Autodesk Inventor part; units mm, degrees
(part 2 of 2)
  line L496 (6.7661, -13.5845) -> (6.8293, -13.6645) construction
  line L497 (6.8293, -13.6645) -> (6.8259, -13.7023) construction
  line L498 (6.8259, -13.7023) -> (6.8218, -13.747) construction
  line L499 (6.8218, -13.747) -> (6.7624, -13.8212) construction
  line L500 (6.7624, -13.8212) -> (6.7246, -13.8227) construction
  line L501 (6.7246, -13.8227) -> (6.4551, -13.8332) construction
  line L502 (6.4551, -13.8332) -> (6.185, -13.8306) construction
  line L503 (6.185, -13.8306) -> (5.9152, -13.8264) construction
  line L504 (5.9152, -13.8264) -> (5.8753, -13.8258) construction
  line L505 (5.8753, -13.8258) -> (5.8359, -13.7944) construction
  line L506 (5.8359, -13.7944) -> (5.7963, -13.7773) construction
  line L507 (5.7963, -13.7773) -> (5.7963, -13.7286) construction
  line L508 (5.7963, -13.7286) -> (5.7963, -13.68) construction
  line L509 (5.7963, -13.68) -> (5.7963, -13.6313) construction
  spline S21 degree 3 poles (5.7963, -12.2084) (6.1054, -12.1913) (6.4145, -12.17) (6.7238, -12.163) (6.7594, -12.1622) (6.8243, -12.2405) (6.8254, -12.2834) (6.8264, -12.324) (6.7627, -12.4009) (6.7252, -12.4023) (6.4526, -12.4122) (6.1794, -12.409) (5.9065, -12.4044) (5.8695, -12.4037) (5.833, -12.3718) (5.7963, -12.3543) (5.7963, -12.3057) (5.7963, -12.257) (5.7963, -12.2084) knots 0 0 0 0 1 1 1 2 2 2 3 3 3 4 4 4 5 5 5 6 6 6 6
  line L510 (5.7963, -12.2084) -> (6.1054, -12.1913) construction
  line L511 (6.1054, -12.1913) -> (6.4145, -12.17) construction
  line L512 (6.4145, -12.17) -> (6.7238, -12.163) construction
  line L513 (6.7238, -12.163) -> (6.7594, -12.1622) construction
  line L514 (6.7594, -12.1622) -> (6.8243, -12.2405) construction
  line L515 (6.8243, -12.2405) -> (6.8254, -12.2834) construction
  line L516 (6.8254, -12.2834) -> (6.8264, -12.324) construction
  line L517 (6.8264, -12.324) -> (6.7627, -12.4009) construction
  line L518 (6.7627, -12.4009) -> (6.7252, -12.4023) construction
  line L519 (6.7252, -12.4023) -> (6.4526, -12.4122) construction
  line L520 (6.4526, -12.4122) -> (6.1794, -12.409) construction
  line L521 (6.1794, -12.409) -> (5.9065, -12.4044) construction
  line L522 (5.9065, -12.4044) -> (5.8695, -12.4037) construction
  line L523 (5.8695, -12.4037) -> (5.833, -12.3718) construction
  line L524 (5.833, -12.3718) -> (5.7963, -12.3543) construction
  line L525 (5.7963, -12.3543) -> (5.7963, -12.3057) construction
  line L526 (5.7963, -12.3057) -> (5.7963, -12.257) construction
  line L527 (5.7963, -12.257) -> (5.7963, -12.2084) construction
  spline S22 degree 3 poles (10.3388, -17.736) (10.3217, -17.43) (10.2998, -17.124) (10.2933, -16.8177) (10.2925, -16.7792) (10.369, -16.7138) (10.4159, -16.7076) (10.4519, -16.7028) (10.5321, -16.7702) (10.5336, -16.8078) (10.5438, -17.0774) (10.541, -17.3475) (10.5363, -17.6174) (10.5356, -17.6573) (10.5027, -17.6965) (10.4848, -17.736) (10.4361, -17.736) (10.3875, -17.736) (10.3388, -17.736) knots 0 0 0 0 1 1 1 2 2 2 3 3 3 4 4 4 5 5 5 6 6 6 6
  line L528 (10.3388, -17.736) -> (10.3217, -17.43) construction
  line L529 (10.3217, -17.43) -> (10.2998, -17.124) construction
  line L530 (10.2998, -17.124) -> (10.2933, -16.8177) construction
  line L531 (10.2933, -16.8177) -> (10.2925, -16.7792) construction
  line L532 (10.2925, -16.7792) -> (10.369, -16.7138) construction
  line L533 (10.369, -16.7138) -> (10.4159, -16.7076) construction
  line L534 (10.4159, -16.7076) -> (10.4519, -16.7028) construction
  line L535 (10.4519, -16.7028) -> (10.5321, -16.7702) construction
  line L536 (10.5321, -16.7702) -> (10.5336, -16.8078) construction
  line L537 (10.5336, -16.8078) -> (10.5438, -17.0774) construction
  line L538 (10.5438, -17.0774) -> (10.541, -17.3475) construction
  line L539 (10.541, -17.3475) -> (10.5363, -17.6174) construction
  line L540 (10.5363, -17.6174) -> (10.5356, -17.6573) construction
  line L541 (10.5356, -17.6573) -> (10.5027, -17.6965) construction
  line L542 (10.5027, -17.6965) -> (10.4848, -17.736) construction
  line L543 (10.4848, -17.736) -> (10.4361, -17.736) construction
  line L544 (10.4361, -17.736) -> (10.3875, -17.736) construction
  line L545 (10.3875, -17.736) -> (10.3388, -17.736) construction
  spline S23 degree 3 poles (8.3868, -9.0888) (8.3978, -9.3955) (8.4126, -9.7023) (8.414, -10.0091) (8.4142, -10.0417) (8.3381, -10.0971) (8.2941, -10.1006) (8.256, -10.1036) (8.1788, -10.0488) (8.1779, -10.0179) (8.1697, -9.7333) (8.1736, -9.4484) (8.1765, -9.1635) (8.1768, -9.1385) (8.1947, -9.1137) (8.2044, -9.0888) (8.2652, -9.0888) (8.326, -9.0888) (8.3868, -9.0888) knots 0 0 0 0 1 1 1 2 2 2 3 3 3 4 4 4 5 5 5 6 6 6 6
  line L546 (8.3868, -9.0888) -> (8.3978, -9.3955) construction
  line L547 (8.3978, -9.3955) -> (8.4126, -9.7023) construction
  line L548 (8.4126, -9.7023) -> (8.414, -10.0091) construction
  line L549 (8.414, -10.0091) -> (8.4142, -10.0417) construction
  line L550 (8.4142, -10.0417) -> (8.3381, -10.0971) construction
  line L551 (8.3381, -10.0971) -> (8.2941, -10.1006) construction
  line L552 (8.2941, -10.1006) -> (8.256, -10.1036) construction
  line L553 (8.256, -10.1036) -> (8.1788, -10.0488) construction
  line L554 (8.1788, -10.0488) -> (8.1779, -10.0179) construction
  line L555 (8.1779, -10.0179) -> (8.1697, -9.7333) construction
  line L556 (8.1697, -9.7333) -> (8.1736, -9.4484) construction
  line L557 (8.1736, -9.4484) -> (8.1765, -9.1635) construction
  line L558 (8.1765, -9.1635) -> (8.1768, -9.1385) construction
  line L559 (8.1768, -9.1385) -> (8.1947, -9.1137) construction
  line L560 (8.1947, -9.1137) -> (8.2044, -9.0888) construction
  line L561 (8.2044, -9.0888) -> (8.2652, -9.0888) construction
  line L562 (8.2652, -9.0888) -> (8.326, -9.0888) construction
  line L563 (8.326, -9.0888) -> (8.3868, -9.0888) construction
  spline S24 degree 3 poles (10.503, -9.0888) (10.5173, -9.2405) (10.5375, -9.392) (10.5443, -9.5441) (10.5507, -9.6893) (10.5531, -9.8362) (10.5362, -9.9799) (10.5307, -10.0262) (10.4583, -10.0646) (10.4165, -10.1066) (10.3733, -10.062) (10.2948, -10.0192) (10.2926, -9.9726) (10.2803, -9.7215) (10.2853, -9.4695) (10.2885, -9.2178) (10.289, -9.1747) (10.3094, -9.1318) (10.3206, -9.0888) (10.3814, -9.0888) (10.4422, -9.0888) (10.503, -9.0888) knots 0 0 0 0 1 1 1 2 2 2 3 3 3 4 4 4 5 5 5 6 6 6 7 7 7 7
  line L564 (10.503, -9.0888) -> (10.5173, -9.2405) construction
  line L565 (10.5173, -9.2405) -> (10.5375, -9.392) construction
  line L566 (10.5375, -9.392) -> (10.5443, -9.5441) construction
  line L567 (10.5443, -9.5441) -> (10.5507, -9.6893) construction
  line L568 (10.5507, -9.6893) -> (10.5531, -9.8362) construction
  line L569 (10.5531, -9.8362) -> (10.5362, -9.9799) construction
  line L570 (10.5362, -9.9799) -> (10.5307, -10.0262) construction
  line L571 (10.5307, -10.0262) -> (10.4583, -10.0646) construction
  line L572 (10.4583, -10.0646) -> (10.4165, -10.1066) construction
  line L573 (10.4165, -10.1066) -> (10.3733, -10.062) construction
  line L574 (10.3733, -10.062) -> (10.2948, -10.0192) construction
  line L575 (10.2948, -10.0192) -> (10.2926, -9.9726) construction
  line L576 (10.2926, -9.9726) -> (10.2803, -9.7215) construction
  line L577 (10.2803, -9.7215) -> (10.2853, -9.4695) construction
  line L578 (10.2853, -9.4695) -> (10.2885, -9.2178) construction
  line L579 (10.2885, -9.2178) -> (10.289, -9.1747) construction
  line L580 (10.289, -9.1747) -> (10.3094, -9.1318) construction
  line L581 (10.3094, -9.1318) -> (10.3206, -9.0888) construction
  line L582 (10.3206, -9.0888) -> (10.3814, -9.0888) construction
  line L583 (10.3814, -9.0888) -> (10.4422, -9.0888) construction
  line L584 (10.4422, -9.0888) -> (10.503, -9.0888) construction
  spline S25 degree 3 poles (14.4435, -13.7955) (14.1371, -13.8063) (13.8306, -13.8209) (13.5241, -13.8221) (13.4913, -13.8222) (13.4356, -13.7462) (13.432, -13.7022) (13.429, -13.6642) (13.4854, -13.5861) (13.5151, -13.5863) (13.8246, -13.5882) (14.1341, -13.6023) (14.4435, -13.6131) (14.4435, -13.6739) (14.4435, -13.7347) (14.4435, -13.7955) knots 0 0 0 0 1 1 1 2 2 2 3 3 3 4 4 4 5 5 5 5
  line L585 (14.4435, -13.7955) -> (14.1371, -13.8063) construction
  line L586 (14.1371, -13.8063) -> (13.8306, -13.8209) construction
  line L587 (13.8306, -13.8209) -> (13.5241, -13.8221) construction
  line L588 (13.5241, -13.8221) -> (13.4913, -13.8222) construction
  line L589 (13.4913, -13.8222) -> (13.4356, -13.7462) construction
  line L590 (13.4356, -13.7462) -> (13.432, -13.7022) construction
  line L591 (13.432, -13.7022) -> (13.429, -13.6642) construction
  line L592 (13.429, -13.6642) -> (13.4854, -13.5861) construction
  line L593 (13.4854, -13.5861) -> (13.5151, -13.5863) construction
  line L594 (13.5151, -13.5863) -> (13.8246, -13.5882) construction
  line L595 (13.8246, -13.5882) -> (14.1341, -13.6023) construction
  line L596 (14.1341, -13.6023) -> (14.4435, -13.6131) construction
  line L597 (14.4435, -13.6131) -> (14.4435, -13.6739) construction
  line L598 (14.4435, -13.6739) -> (14.4435, -13.7347) construction
  line L599 (14.4435, -13.7347) -> (14.4435, -13.7955) construction
  spline S26 degree 3 poles (14.4435, -15.1455) (14.1369, -15.1566) (13.8303, -15.1712) (13.5236, -15.1734) (13.4909, -15.1737) (13.4316, -15.1015) (13.4318, -15.0632) (13.432, -15.0191) (13.4847, -14.937) (13.5144, -14.9371) (13.8242, -14.9382) (14.1338, -14.9525) (14.4435, -14.9631) (14.4435, -15.0239) (14.4435, -15.0847) (14.4435, -15.1455) knots 0 0 0 0 1 1 1 2 2 2 3 3 3 4 4 4 5 5 5 5
  line L600 (14.4435, -15.1455) -> (14.1369, -15.1566) construction
  line L601 (14.1369, -15.1566) -> (13.8303, -15.1712) construction
  line L602 (13.8303, -15.1712) -> (13.5236, -15.1734) construction
  line L603 (13.5236, -15.1734) -> (13.4909, -15.1737) construction
  line L604 (13.4909, -15.1737) -> (13.4316, -15.1015) construction
  line L605 (13.4316, -15.1015) -> (13.4318, -15.0632) construction
  line L606 (13.4318, -15.0632) -> (13.432, -15.0191) construction
  line L607 (13.432, -15.0191) -> (13.4847, -14.937) construction
  line L608 (13.4847, -14.937) -> (13.5144, -14.9371) construction
  line L609 (13.5144, -14.9371) -> (13.8242, -14.9382) construction
  line L610 (13.8242, -14.9382) -> (14.1338, -14.9525) construction
  line L611 (14.1338, -14.9525) -> (14.4435, -14.9631) construction
  line L612 (14.4435, -14.9631) -> (14.4435, -15.0239) construction
  line L613 (14.4435, -15.0239) -> (14.4435, -15.0847) construction
  line L614 (14.4435, -15.0847) -> (14.4435, -15.1455) construction
  spline S27 degree 3 poles (14.4435, -12.3726) (14.2342, -12.3858) (14.0249, -12.4009) (13.8154, -12.4116) (13.7278, -12.416) (13.6362, -12.4254) (13.5533, -12.4049) (13.5037, -12.3926) (13.4674, -12.3265) (13.4251, -12.2846) (13.4703, -12.2418) (13.5137, -12.1642) (13.5608, -12.1619) (13.8117, -12.1497) (14.0635, -12.1548) (14.3149, -12.158) (14.3579, -12.1586) (14.4006, -12.1789) (14.4435, -12.1901) (14.4435, -12.2509) (14.4435, -12.3117) (14.4435, -12.3726) knots 0 0 0 0 1 1 1 2 2 2 3 3 3 4 4 4 5 5 5 6 6 6 7 7 7 7
  line L615 (14.4435, -12.3726) -> (14.2342, -12.3858) construction
  line L616 (14.2342, -12.3858) -> (14.0249, -12.4009) construction
  line L617 (14.0249, -12.4009) -> (13.8154, -12.4116) construction
  line L618 (13.8154, -12.4116) -> (13.7278, -12.416) construction
  line L619 (13.7278, -12.416) -> (13.6362, -12.4254) construction
  line L620 (13.6362, -12.4254) -> (13.5533, -12.4049) construction
  line L621 (13.5533, -12.4049) -> (13.5037, -12.3926) construction
  line L622 (13.5037, -12.3926) -> (13.4674, -12.3265) construction
  line L623 (13.4674, -12.3265) -> (13.4251, -12.2846) construction
  line L624 (13.4251, -12.2846) -> (13.4703, -12.2418) construction
  line L625 (13.4703, -12.2418) -> (13.5137, -12.1642) construction
  line L626 (13.5137, -12.1642) -> (13.5608, -12.1619) construction
  line L627 (13.5608, -12.1619) -> (13.8117, -12.1497) construction
  line L628 (13.8117, -12.1497) -> (14.0635, -12.1548) construction
  line L629 (14.0635, -12.1548) -> (14.3149, -12.158) construction
  line L630 (14.3149, -12.158) -> (14.3579, -12.1586) construction
  line L631 (14.3579, -12.1586) -> (14.4006, -12.1789) construction
  line L632 (14.4006, -12.1789) -> (14.4435, -12.1901) construction
  line L633 (14.4435, -12.1901) -> (14.4435, -12.2509) construction
  line L634 (14.4435, -12.2509) -> (14.4435, -12.3117) construction
  line L635 (14.4435, -12.3117) -> (14.4435, -12.3726) construction
  spline S28 degree 3 poles (7.9415, -15.0093) (7.9425, -15.1487) (8.0504, -15.2573) (8.1887, -15.2582) (8.3296, -15.2591) (8.4452, -15.1449) (8.444, -15.006) (8.4428, -14.863) (8.3326, -14.7578) (8.1855, -14.7592) (8.0453, -14.7605) (7.9405, -14.8679) (7.9415, -15.0093) knots 0 0 0 0 1 1 1 2 2 2 3 3 3 4 4 4 4
  line L636 (7.9415, -15.0093) -> (7.9425, -15.1487) construction
  line L637 (7.9425, -15.1487) -> (8.0504, -15.2573) construction
  line L638 (8.0504, -15.2573) -> (8.1887, -15.2582) construction
  line L639 (8.1887, -15.2582) -> (8.3296, -15.2591) construction
  line L640 (8.3296, -15.2591) -> (8.4452, -15.1449) construction
  line L641 (8.4452, -15.1449) -> (8.444, -15.006) construction
  line L642 (8.444, -15.006) -> (8.4428, -14.863) construction
  line L643 (8.4428, -14.863) -> (8.3326, -14.7578) construction
  line L644 (8.3326, -14.7578) -> (8.1855, -14.7592) construction
  line L645 (8.1855, -14.7592) -> (8.0453, -14.7605) construction
  line L646 (8.0453, -14.7605) -> (7.9405, -14.8679) construction
  line L647 (7.9405, -14.8679) -> (7.9415, -15.0093) construction
  spline S29 degree 3 poles (9.9835, -11.9696) (9.5672, -11.9696) (9.1509, -11.9714) (8.7347, -11.9679) (8.6601, -11.9673) (8.6371, -11.9855) (8.6374, -12.0631) (8.6403, -12.8865) (8.6405, -13.7099) (8.6374, -14.5333) (8.6371, -14.6168) (8.6587, -14.6393) (8.7426, -14.639) (9.572, -14.6358) (10.4015, -14.636) (11.231, -14.6386) (11.3057, -14.6389) (11.3291, -14.6213) (11.3289, -14.5439) (11.3261, -13.7175) (11.326, -12.8911) (11.3286, -12.0646) (11.3288, -11.9885) (11.3082, -11.967) (11.2322, -11.9676) (10.816, -11.9711) (10.3997, -11.9693) (9.9835, -11.9696) knots 0 0 0 0 1 1 1 2 2 2 3 3 3 4 4 4 5 5 5 6 6 6 7 7 7 8 8 8 9 9 9 9
  line L648 (9.9835, -11.9696) -> (9.5672, -11.9696) construction
  line L649 (9.5672, -11.9696) -> (9.1509, -11.9714) construction
  line L650 (9.1509, -11.9714) -> (8.7347, -11.9679) construction
  line L651 (8.7347, -11.9679) -> (8.6601, -11.9673) construction
  line L652 (8.6601, -11.9673) -> (8.6371, -11.9855) construction
  line L653 (8.6371, -11.9855) -> (8.6374, -12.0631) construction
  line L654 (8.6374, -12.0631) -> (8.6403, -12.8865) construction
  line L655 (8.6403, -12.8865) -> (8.6405, -13.7099) construction
  line L656 (8.6405, -13.7099) -> (8.6374, -14.5333) construction
  line L657 (8.6374, -14.5333) -> (8.6371, -14.6168) construction
  line L658 (8.6371, -14.6168) -> (8.6587, -14.6393) construction
  line L659 (8.6587, -14.6393) -> (8.7426, -14.639) construction
  line L660 (8.7426, -14.639) -> (9.572, -14.6358) construction
  line L661 (9.572, -14.6358) -> (10.4015, -14.636) construction
  line L662 (10.4015, -14.636) -> (11.231, -14.6386) construction
  line L663 (11.231, -14.6386) -> (11.3057, -14.6389) construction
  line L664 (11.3057, -14.6389) -> (11.3291, -14.6213) construction
  line L665 (11.3291, -14.6213) -> (11.3289, -14.5439) construction
  line L666 (11.3289, -14.5439) -> (11.3261, -13.7175) construction
  line L667 (11.3261, -13.7175) -> (11.326, -12.8911) construction
  line L668 (11.326, -12.8911) -> (11.3286, -12.0646) construction
  line L669 (11.3286, -12.0646) -> (11.3288, -11.9885) construction
  line L670 (11.3288, -11.9885) -> (11.3082, -11.967) construction
  line L671 (11.3082, -11.967) -> (11.2322, -11.9676) construction
  line L672 (11.2322, -11.9676) -> (10.816, -11.9711) construction
  line L673 (10.816, -11.9711) -> (10.3997, -11.9693) construction
  line L674 (10.3997, -11.9693) -> (9.9835, -11.9696) construction
  spline S30 degree 3 poles (10.0561, -10.4237) (10.7462, -10.4238) (11.4363, -10.4237) (12.1264, -10.4238) (12.6095, -10.4239) (12.9621, -10.7733) (12.9623, -11.2548) (12.9629, -12.6289) (12.9628, -14.0031) (12.9623, -15.3772) (12.9621, -15.853) (12.6241, -16.2096) (12.1487, -16.2114) (10.7594, -16.2167) (9.37, -16.2169) (7.9807, -16.211) (7.5042, -16.209) (7.1679, -15.8523) (7.1678, -15.3765) (7.1677, -14.0206) (7.1678, -12.6648) (7.1679, -11.3089) (7.1679, -10.7543) (7.4971, -10.4237) (8.0497, -10.4236) (8.7185, -10.4235) (9.3873, -10.4236) (10.0561, -10.4237) knots 0 0 0 0 1 1 1 2 2 2 3 3 3 4 4 4 5 5 5 6 6 6 7 7 7 8 8 8 9 9 9 9
  line L675 (10.0561, -10.4237) -> (10.7462, -10.4238) construction
  line L676 (10.7462, -10.4238) -> (11.4363, -10.4237) construction
  line L677 (11.4363, -10.4237) -> (12.1264, -10.4238) construction
  line L678 (12.1264, -10.4238) -> (12.6095, -10.4239) construction
  line L679 (12.6095, -10.4239) -> (12.9621, -10.7733) construction
  line L680 (12.9621, -10.7733) -> (12.9623, -11.2548) construction
  line L681 (12.9623, -11.2548) -> (12.9629, -12.6289) construction
  line L682 (12.9629, -12.6289) -> (12.9628, -14.0031) construction
  line L683 (12.9628, -14.0031) -> (12.9623, -15.3772) construction
  line L684 (12.9623, -15.3772) -> (12.9621, -15.853) construction
  line L685 (12.9621, -15.853) -> (12.6241, -16.2096) construction
  line L686 (12.6241, -16.2096) -> (12.1487, -16.2114) construction
  line L687 (12.1487, -16.2114) -> (10.7594, -16.2167) construction
  line L688 (10.7594, -16.2167) -> (9.37, -16.2169) construction
  line L689 (9.37, -16.2169) -> (7.9807, -16.211) construction
  line L690 (7.9807, -16.211) -> (7.5042, -16.209) construction
  line L691 (7.5042, -16.209) -> (7.1679, -15.8523) construction
  line L692 (7.1679, -15.8523) -> (7.1678, -15.3765) construction
  line L693 (7.1678, -15.3765) -> (7.1677, -14.0206) construction
  line L694 (7.1677, -14.0206) -> (7.1678, -12.6648) construction
  line L695 (7.1678, -12.6648) -> (7.1679, -11.3089) construction
  line L696 (7.1679, -11.3089) -> (7.1679, -10.7543) construction
  line L697 (7.1679, -10.7543) -> (7.4971, -10.4237) construction
  line L698 (7.4971, -10.4237) -> (8.0497, -10.4236) construction
  line L699 (8.0497, -10.4236) -> (8.7185, -10.4235) construction
  line L700 (8.7185, -10.4235) -> (9.3873, -10.4236) construction
  line L701 (9.3873, -10.4236) -> (10.0561, -10.4237) construction
  spline S31 degree 3 poles (-4.7644, 1.7423) (-2.9929, 1.753) (-1.4236, 1.1881) (-0.0506, 0.0741) (0.7591, -0.5829) (1.4031, -1.3793) (1.9078, -2.2904) (1.9458, -2.3589) (1.944, -2.3927) (1.873, -2.4384) (1.5083, -2.6729) (1.1477, -2.9138) (0.7857, -3.1525) (0.698, -3.2103) (0.699, -3.2099) (0.643, -3.1163) (-0.1092, -1.8584) (-1.1564, -0.9472) (-2.5312, -0.4246) (-3.0361, -0.2326) (-3.5589, -0.1101) (-4.099, -0.0778) (-6.3771, 0.0587) (-8.161, -0.8436) (-9.5067, -2.6607) (-9.56, -2.7327) (-9.6087, -2.8082) (-9.6569, -2.8837) (-9.6813, -2.922) (-9.7032, -2.924) (-9.7377, -2.8956) (-10.1326, -2.571) (-10.5278, -2.2466) (-10.9243, -1.9239) (-10.9693, -1.8874) (-10.9566, -1.8588) (-10.9317, -1.8198) (-10.4723, -1.099) (-9.918, -0.4616) (-9.2556, 0.0797) (-8.3533, 0.8171) (-7.3362, 1.3217) (-6.1975, 1.5758) (-5.7261, 1.6809) (-5.2482, 1.7362) (-4.7644, 1.7423) knots 0 0 0 0 1 1 1 2 2 2 3 3 3 4 4 4 5 5 5 6 6 6 7 7 7 8 8 8 9 9 9 10 10 10 11 11 11 12 12 12 13 13 13 14 14 14 15 15 15 15
  line L702 (-4.7644, 1.7423) -> (-2.9929, 1.753) construction
  line L703 (-2.9929, 1.753) -> (-1.4236, 1.1881) construction
  line L704 (-1.4236, 1.1881) -> (-0.0506, 0.0741) construction
  line L705 (-0.0506, 0.0741) -> (0.7591, -0.5829) construction
  line L706 (0.7591, -0.5829) -> (1.4031, -1.3793) construction
  line L707 (1.4031, -1.3793) -> (1.9078, -2.2904) construction
  line L708 (1.9078, -2.2904) -> (1.9458, -2.3589) construction
  line L709 (1.9458, -2.3589) -> (1.944, -2.3927) construction
  line L710 (1.944, -2.3927) -> (1.873, -2.4384) construction
  line L711 (1.873, -2.4384) -> (1.5083, -2.6729) construction
  line L712 (1.5083, -2.6729) -> (1.1477, -2.9138) construction
  line L713 (1.1477, -2.9138) -> (0.7857, -3.1525) construction
  line L714 (0.7857, -3.1525) -> (0.698, -3.2103) construction
  line L715 (0.698, -3.2103) -> (0.699, -3.2099) construction
  line L716 (0.699, -3.2099) -> (0.643, -3.1163) construction
  line L717 (0.643, -3.1163) -> (-0.1092, -1.8584) construction
  line L718 (-0.1092, -1.8584) -> (-1.1564, -0.9472) construction
  line L719 (-1.1564, -0.9472) -> (-2.5312, -0.4246) construction
  line L720 (-2.5312, -0.4246) -> (-3.0361, -0.2326) construction
  line L721 (-3.0361, -0.2326) -> (-3.5589, -0.1101) construction
  line L722 (-3.5589, -0.1101) -> (-4.099, -0.0778) construction
  line L723 (-4.099, -0.0778) -> (-6.3771, 0.0587) construction
  line L724 (-6.3771, 0.0587) -> (-8.161, -0.8436) construction
  line L725 (-8.161, -0.8436) -> (-9.5067, -2.6607) construction
  line L726 (-9.5067, -2.6607) -> (-9.56, -2.7327) construction
  line L727 (-9.56, -2.7327) -> (-9.6087, -2.8082) construction
  line L728 (-9.6087, -2.8082) -> (-9.6569, -2.8837) construction
  line L729 (-9.6569, -2.8837) -> (-9.6813, -2.922) construction
  line L730 (-9.6813, -2.922) -> (-9.7032, -2.924) construction
  line L731 (-9.7032, -2.924) -> (-9.7377, -2.8956) construction
  line L732 (-9.7377, -2.8956) -> (-10.1326, -2.571) construction
  line L733 (-10.1326, -2.571) -> (-10.5278, -2.2466) construction
  line L734 (-10.5278, -2.2466) -> (-10.9243, -1.9239) construction
  line L735 (-10.9243, -1.9239) -> (-10.9693, -1.8874) construction
  line L736 (-10.9693, -1.8874) -> (-10.9566, -1.8588) construction
  line L737 (-10.9566, -1.8588) -> (-10.9317, -1.8198) construction
  line L738 (-10.9317, -1.8198) -> (-10.4723, -1.099) construction
  line L739 (-10.4723, -1.099) -> (-9.918, -0.4616) construction
  line L740 (-9.918, -0.4616) -> (-9.2556, 0.0797) construction
  line L741 (-9.2556, 0.0797) -> (-8.3533, 0.8171) construction
  line L742 (-8.3533, 0.8171) -> (-7.3362, 1.3217) construction
  line L743 (-7.3362, 1.3217) -> (-6.1975, 1.5758) construction
  line L744 (-6.1975, 1.5758) -> (-5.7261, 1.6809) construction
  line L745 (-5.7261, 1.6809) -> (-5.2482, 1.7362) construction
  line L746 (-5.2482, 1.7362) -> (-4.7644, 1.7423) construction
  spline S32 degree 3 poles (-4.6061, -2.5961) (-5.9351, -2.6535) (-6.9655, -3.2452) (-7.7141, -4.3402) (-7.7762, -4.431) (-7.7746, -4.4316) (-7.8619, -4.36) (-8.1147, -4.1526) (-8.3671, -3.9446) (-8.6213, -3.739) (-8.6649, -3.7037) (-8.6771, -3.6769) (-8.6418, -3.6264) (-7.8661, -2.5153) (-6.827, -1.7781) (-5.4899, -1.5435) (-3.5634, -1.2055) (-1.9737, -1.8393) (-0.7247, -3.3369) (-0.6134, -3.4704) (-0.5228, -3.6209) (-0.4197, -3.7615) (-0.3781, -3.8183) (-0.3802, -3.8517) (-0.4447, -3.8929) (-0.7019, -4.0572) (-0.9571, -4.2247) (-1.2087, -4.3972) (-1.28, -4.4461) (-1.3091, -4.4312) (-1.3534, -4.3643) (-1.8925, -3.5488) (-2.6253, -2.9925) (-3.5702, -2.7264) (-3.9075, -2.6314) (-4.2525, -2.5872) (-4.6061, -2.5961) knots 0 0 0 0 1 1 1 2 2 2 3 3 3 4 4 4 5 5 5 6 6 6 7 7 7 8 8 8 9 9 9 10 10 10 11 11 11 12 12 12 12
  line L747 (-4.6061, -2.5961) -> (-5.9351, -2.6535) construction
  line L748 (-5.9351, -2.6535) -> (-6.9655, -3.2452) construction
  line L749 (-6.9655, -3.2452) -> (-7.7141, -4.3402) construction
  line L750 (-7.7141, -4.3402) -> (-7.7762, -4.431) construction
  line L751 (-7.7762, -4.431) -> (-7.7746, -4.4316) construction
  line L752 (-7.7746, -4.4316) -> (-7.8619, -4.36) construction
  line L753 (-7.8619, -4.36) -> (-8.1147, -4.1526) construction
  line L754 (-8.1147, -4.1526) -> (-8.3671, -3.9446) construction
  line L755 (-8.3671, -3.9446) -> (-8.6213, -3.739) construction
  line L756 (-8.6213, -3.739) -> (-8.6649, -3.7037) construction
  line L757 (-8.6649, -3.7037) -> (-8.6771, -3.6769) construction
  line L758 (-8.6771, -3.6769) -> (-8.6418, -3.6264) construction
  line L759 (-8.6418, -3.6264) -> (-7.8661, -2.5153) construction
  line L760 (-7.8661, -2.5153) -> (-6.827, -1.7781) construction
  line L761 (-6.827, -1.7781) -> (-5.4899, -1.5435) construction
  line L762 (-5.4899, -1.5435) -> (-3.5634, -1.2055) construction
  line L763 (-3.5634, -1.2055) -> (-1.9737, -1.8393) construction
  line L764 (-1.9737, -1.8393) -> (-0.7247, -3.3369) construction
  line L765 (-0.7247, -3.3369) -> (-0.6134, -3.4704) construction
  line L766 (-0.6134, -3.4704) -> (-0.5228, -3.6209) construction
  line L767 (-0.5228, -3.6209) -> (-0.4197, -3.7615) construction
  line L768 (-0.4197, -3.7615) -> (-0.3781, -3.8183) construction
  line L769 (-0.3781, -3.8183) -> (-0.3802, -3.8517) construction
  line L770 (-0.3802, -3.8517) -> (-0.4447, -3.8929) construction
  line L771 (-0.4447, -3.8929) -> (-0.7019, -4.0572) construction
  line L772 (-0.7019, -4.0572) -> (-0.9571, -4.2247) construction
  line L773 (-0.9571, -4.2247) -> (-1.2087, -4.3972) construction
  line L774 (-1.2087, -4.3972) -> (-1.28, -4.4461) construction
  line L775 (-1.28, -4.4461) -> (-1.3091, -4.4312) construction
  line L776 (-1.3091, -4.4312) -> (-1.3534, -4.3643) construction
  line L777 (-1.3534, -4.3643) -> (-1.8925, -3.5488) construction
  line L778 (-1.8925, -3.5488) -> (-2.6253, -2.9925) construction
  line L779 (-2.6253, -2.9925) -> (-3.5702, -2.7264) construction
  line L780 (-3.5702, -2.7264) -> (-3.9075, -2.6314) construction
  line L781 (-3.9075, -2.6314) -> (-4.2525, -2.5872) construction
  line L782 (-4.2525, -2.5872) -> (-4.6061, -2.5961) construction
  spline S33 degree 3 poles (-4.6398, -3.6243) (-3.6408, -3.6412) (-2.8604, -4.0349) (-2.264, -4.7999) (-2.2209, -4.8553) (-2.2306, -4.8813) (-2.2861, -4.917) (-2.5, -5.0543) (-2.7124, -5.1942) (-2.9226, -5.3371) (-2.9773, -5.3744) (-3.0079, -5.3722) (-3.0539, -5.3211) (-3.4137, -4.9205) (-3.8614, -4.6784) (-4.3992, -4.6388) (-5.1565, -4.5831) (-5.7606, -4.8809) (-6.2183, -5.4823) (-6.2835, -5.568) (-6.2814, -5.5687) (-6.3628, -5.5018) (-6.5573, -5.3419) (-6.7513, -5.1813) (-6.9477, -5.0236) (-6.9906, -4.9891) (-6.9976, -4.9617) (-6.9652, -4.9158) (-6.4787, -4.225) (-5.8287, -3.7922) (-4.9875, -3.6623) (-4.8635, -3.6431) (-4.7378, -3.6348) (-4.6398, -3.6243) knots 0 0 0 0 1 1 1 2 2 2 3 3 3 4 4 4 5 5 5 6 6 6 7 7 7 8 8 8 9 9 9 10 10 10 11 11 11 11
  line L783 (-4.6398, -3.6243) -> (-3.6408, -3.6412) construction
  line L784 (-3.6408, -3.6412) -> (-2.8604, -4.0349) construction
  line L785 (-2.8604, -4.0349) -> (-2.264, -4.7999) construction
  line L786 (-2.264, -4.7999) -> (-2.2209, -4.8553) construction
  line L787 (-2.2209, -4.8553) -> (-2.2306, -4.8813) construction
  line L788 (-2.2306, -4.8813) -> (-2.2861, -4.917) construction
  line L789 (-2.2861, -4.917) -> (-2.5, -5.0543) construction
  line L790 (-2.5, -5.0543) -> (-2.7124, -5.1942) construction
  line L791 (-2.7124, -5.1942) -> (-2.9226, -5.3371) construction
  line L792 (-2.9226, -5.3371) -> (-2.9773, -5.3744) construction
  line L793 (-2.9773, -5.3744) -> (-3.0079, -5.3722) construction
  line L794 (-3.0079, -5.3722) -> (-3.0539, -5.3211) construction
  line L795 (-3.0539, -5.3211) -> (-3.4137, -4.9205) construction
  line L796 (-3.4137, -4.9205) -> (-3.8614, -4.6784) construction
  line L797 (-3.8614, -4.6784) -> (-4.3992, -4.6388) construction
  line L798 (-4.3992, -4.6388) -> (-5.1565, -4.5831) construction
  line L799 (-5.1565, -4.5831) -> (-5.7606, -4.8809) construction
  line L800 (-5.7606, -4.8809) -> (-6.2183, -5.4823) construction
  line L801 (-6.2183, -5.4823) -> (-6.2835, -5.568) construction
  line L802 (-6.2835, -5.568) -> (-6.2814, -5.5687) construction
  line L803 (-6.2814, -5.5687) -> (-6.3628, -5.5018) construction
  line L804 (-6.3628, -5.5018) -> (-6.5573, -5.3419) construction
  line L805 (-6.5573, -5.3419) -> (-6.7513, -5.1813) construction
  line L806 (-6.7513, -5.1813) -> (-6.9477, -5.0236) construction
  line L807 (-6.9477, -5.0236) -> (-6.9906, -4.9891) construction
  line L808 (-6.9906, -4.9891) -> (-6.9976, -4.9617) construction
  line L809 (-6.9976, -4.9617) -> (-6.9652, -4.9158) construction
  line L810 (-6.9652, -4.9158) -> (-6.4787, -4.225) construction
  line L811 (-6.4787, -4.225) -> (-5.8287, -3.7922) construction
  line L812 (-5.8287, -3.7922) -> (-4.9875, -3.6623) construction
  line L813 (-4.9875, -3.6623) -> (-4.8635, -3.6431) construction
  line L814 (-4.8635, -3.6431) -> (-4.7378, -3.6348) construction
  line L815 (-4.7378, -3.6348) -> (-4.6398, -3.6243) construction
  spline S34 degree 3 poles (-4.5886, -7.8848) (-5.2743, -7.8921) (-5.8234, -7.3692) (-5.831, -6.7016) (-5.8385, -6.0478) (-5.2922, -5.5069) (-4.6186, -5.5013) (-3.9385, -5.4956) (-3.3883, -6.0174) (-3.382, -6.6742) (-3.3756, -7.3431) (-3.9083, -7.8776) (-4.5886, -7.8848) knots 0 0 0 0 1 1 1 2 2 2 3 3 3 4 4 4 4
  line L816 (-4.5886, -7.8848) -> (-5.2743, -7.8921) construction
  line L817 (-5.2743, -7.8921) -> (-5.8234, -7.3692) construction
  line L818 (-5.8234, -7.3692) -> (-5.831, -6.7016) construction
  line L819 (-5.831, -6.7016) -> (-5.8385, -6.0478) construction
  line L820 (-5.8385, -6.0478) -> (-5.2922, -5.5069) construction
  line L821 (-5.2922, -5.5069) -> (-4.6186, -5.5013) construction
  line L822 (-4.6186, -5.5013) -> (-3.9385, -5.4956) construction
  line L823 (-3.9385, -5.4956) -> (-3.3883, -6.0174) construction
  line L824 (-3.3883, -6.0174) -> (-3.382, -6.6742) construction
  line L825 (-3.382, -6.6742) -> (-3.3756, -7.3431) construction
  line L826 (-3.3756, -7.3431) -> (-3.9083, -7.8776) construction
  line L827 (-3.9083, -7.8776) -> (-4.5886, -7.8848) construction
  point P0 (0, 0)
  constraints: 67 other
extrude "Extrusion3" cut sketch "Sketch4" against normal blind 1.5
body "Solid1"
